Autodesk Fusion 360 part; units mm, degrees
(part 16 of 24)
  line L1627 (7.7089, 53.5468) -> (7.5354, 53.8714)
  line L1628 (4.6355, 51.6255) -> (4.6355, 48.2096)
  arc A4575 (6.3346, 55.2923) -> (6.1582, 55.0284) centre (6.2464, 55.1604) ccw
  line L1629 (6.2464, 55.1604) -> (5.9218, 55.3339)
  arc A4576 (7.8555, 53.6075) -> (7.5622, 53.486) centre (7.7088, 53.5468) ccw
  arc A4577 (7.22, 54.5627) -> (6.9746, 54.3613) centre (7.0973, 54.462) ccw
  line L1630 (5.9218, 55.3339) -> (5.5817, 55.4747)
  arc A4578 (5.6424, 55.6214) -> (5.5209, 55.3281) centre (5.5816, 55.4748) ccw
  arc A4579 (6.6407, 48.7982) -> (6.4643, 49.0621) centre (6.5525, 48.9301) ccw
  arc A4580 (7.4628, 54.2657) -> (7.1988, 54.0893) centre (7.3308, 54.1775) ccw
  arc A4581 (70.8706, 40.7824) -> (70.8706, 40.4649) centre (70.8706, 40.6237) ccw
  arc A4582 (70.2126, 40.4602) -> (70.4372, 40.2356) centre (70.3249, 40.3479) ccw
  arc A4583 (8.0017, 53.2528) -> (7.6978, 53.1606) centre (7.8497, 53.2067) ccw
  line L1631 (6.5525, 54.9558) -> (6.2464, 55.1604)
  line L1632 (7.5354, 53.8714) -> (7.3308, 54.1775)
  arc A4584 (7.8934, 52.2449) -> (8.2093, 52.2761) centre (8.0514, 52.2605) ccw
  arc A4585 (6.1582, 48.8576) -> (6.3346, 48.5936) centre (6.2464, 48.7256) ccw
  arc A4586 (72.0706, 39.9679) -> (72.2951, 40.1924) centre (72.1829, 40.0802) ccw
  arc A4587 (8.1123, 52.8854) -> (7.8009, 52.8235) centre (7.9566, 52.8545) ccw
  line L1633 (70.8706, 40.6237) -> (70.4098, 40.4328)
  arc A4588 (6.7363, 54.5996) -> (6.9377, 54.845) centre (6.837, 54.7223) ccw
  line L1634 (8.0284, 52.4934) -> (7.9566, 52.8544)
  arc A4589 (6.9377, 49.041) -> (6.7363, 49.2864) centre (6.837, 49.1637) ccw
  arc A4590 (70.5221, 40.3206) -> (70.2976, 40.5451) centre (70.4099, 40.4329) ccw
  arc A4591 (8.1864, 52.5089) -> (7.8704, 52.4778) centre (8.0284, 52.4934) ccw
  arc A4592 (7.5689, 53.4719) -> (7.8489, 53.6216) centre (7.7089, 53.5468) ccw
  arc A4593 (7.7031, 53.1459) -> (7.9964, 53.2674) centre (7.8498, 53.2067) ccw
  line L1635 (5.5817, 55.4747) -> (5.415, 55.5253)
  arc A4594 (6.9493, 54.8346) -> (6.7248, 54.6101) centre (6.8371, 54.7224) ccw
  arc A4595 (72.2149, 39.1206) -> (72.5324, 39.1206) centre (72.3736, 39.1206) ccw
  arc A4596 (5.9825, 48.4055) -> (5.861, 48.6988) centre (5.9218, 48.5522) ccw
  arc A4597 (7.8727, 52.4624) -> (8.1841, 52.5244) centre (8.0284, 52.4934) ccw
  arc A4598 (5.9966, 55.4739) -> (5.8469, 55.1939) centre (5.9217, 55.3339) ccw
  line L1636 (8.0514, 52.2605) -> (8.0284, 52.4934)
  arc A4599 (5.861, 55.1872) -> (5.9825, 55.4805) centre (5.9218, 55.3338) ccw
  arc A4600 (70.9314, 40.477) -> (70.8099, 40.7704) centre (70.8706, 40.6237) ccw
  line L1637 (5.415, 55.5253) -> (79.548, 55.5253)
  arc A4601 (5.5356, 55.3228) -> (5.6278, 55.6267) centre (5.5817, 55.4748) ccw
  arc A4602 (7.5622, 50.4) -> (7.8555, 50.2785) centre (7.7088, 50.3392) ccw
  line L1638 (71.3694, 40.6237) -> (70.8706, 40.6237)
  line L1639 (7.7089, 50.3392) -> (7.8497, 50.6793)
  line L1640 (7.3308, 54.1775) -> (7.0973, 54.462)
  line L1641 (72.3737, 39.1206) -> (72.3737, 39.6194)
  arc A4603 (72.5324, 39.6194) -> (72.2149, 39.6194) centre (72.3736, 39.6194) ccw
  line L1642 (6.5525, 48.9302) -> (6.837, 49.1637)
  arc A4604 (4.6355, 52.4192) -> (4.6355, 52.1017) centre (4.6355, 52.2604) ccw
  line L1643 (7.0973, 54.462) -> (6.837, 54.7223)
  arc A4605 (79.548, 55.3666) -> (79.548, 55.684) centre (79.548, 55.5253) ccw
  arc A4606 (7.1988, 49.7967) -> (7.4628, 49.6203) centre (7.3308, 49.7085) ccw
  line L1644 (72.3737, 39.6194) -> (72.1828, 40.0802)
  arc A4607 (7.8047, 52.8083) -> (8.1085, 52.9005) centre (7.9566, 52.8544) ccw
  arc A4608 (72.3295, 40.1409) -> (72.0362, 40.0194) centre (72.1829, 40.0802) ccw
  line L1645 (52.2859, 37.4845) -> (52.2859, 38.2029)
  arc A4609 (52.4446, 38.2029) -> (52.1271, 38.2029) centre (52.2858, 38.2029) ccw
  line L1646 (52.2859, 38.2029) -> (52.4751, 38.3921)
  arc A4610 (51.9362, 40.2012) -> (51.8147, 40.4946) centre (51.8755, 40.3479) ccw
  arc A4611 (50.0723, 36.5018) -> (50.2968, 36.7264) centre (50.1845, 36.6141) ccw
  arc A4612 (6.1716, 55.0203) -> (6.3212, 55.3004) centre (6.2464, 55.1604) ccw
  arc A4613 (71.7694, 40.2862) -> (71.8909, 40.5795) centre (71.8302, 40.4329) ccw
  arc A4614 (52.1271, 37.4845) -> (52.4446, 37.4845) centre (52.2858, 37.4845) ccw
  line L1647 (50.9029, 39.5859) -> (50.1845, 39.5859)
  line L1648 (52.4751, 38.3921) -> (70.3249, 38.3921)
  arc A4615 (70.3249, 38.2334) -> (70.3249, 38.5508) centre (70.3249, 38.3921) ccw
  arc A4616 (52.4751, 38.5508) -> (52.4751, 38.2334) centre (52.4751, 38.3921) ccw
  line L1649 (72.1828, 38.6598) -> (72.3737, 39.1206)
  line L1650 (71.3694, 38.1163) -> (71.8302, 38.3072)
  arc A4617 (50.1845, 36.7728) -> (50.1845, 36.4554) centre (50.1845, 36.6141) ccw
  arc A4618 (52.5873, 38.2798) -> (52.3628, 38.5044) centre (52.4751, 38.3921) ccw
  arc A4619 (52.3982, 37.3723) -> (52.1736, 37.5968) centre (52.2859, 37.4846) ccw
  arc A4620 (51.6283, 40.0868) -> (51.4038, 40.3113) centre (51.516, 40.199) ccw
  arc A4621 (52.1736, 38.3152) -> (52.3982, 38.0907) centre (52.2859, 38.203) ccw
  arc A4622 (70.4372, 38.5044) -> (70.2126, 38.2798) centre (70.3249, 38.3921) ccw
  arc A4623 (51.4155, 36.4554) -> (51.4155, 36.7728) centre (51.4155, 36.6141) ccw
  arc A4624 (49.4264, 37.5968) -> (49.2018, 37.3723) centre (49.3141, 37.4846) ccw
  line L1651 (70.4098, 38.3072) -> (70.8706, 38.1163)
  line L1652 (50.1845, 36.6141) -> (51.4155, 36.6141)
  arc A4625 (70.4706, 38.4538) -> (70.3491, 38.1605) centre (70.4099, 38.3072) ccw
  arc A4626 (70.8099, 37.9696) -> (70.9314, 38.263) centre (70.8706, 38.1163) ccw
  arc A4627 (50.7907, 39.6982) -> (51.0152, 39.4736) centre (50.903, 39.5859) ccw
  line L1653 (53.34, 17.78) -> (53.34, 19.2405)
  line L1654 (53.34, 19.2405) -> (53.34, 17.78)
  line L1655 (71.8302, 40.4328) -> (71.3694, 40.6237)
  line L1656 (51.5161, 40.199) -> (51.241, 39.9239)
  arc A4628 (71.4301, 40.7704) -> (71.3086, 40.477) centre (71.3693, 40.6237) ccw
  line L1657 (7.9566, 52.8544) -> (7.8497, 53.2067)
  arc A4629 (70.8706, 38.2751) -> (70.8706, 37.9576) centre (70.8706, 38.1164) ccw
  arc A4630 (72.2951, 38.5476) -> (72.0706, 38.7721) centre (72.1829, 38.6599) ccw
  line L1658 (51.8755, 40.3479) -> (51.5161, 40.199)
  line L1659 (70.8706, 38.1163) -> (71.3694, 38.1163)
  line L1660 (7.8497, 53.2067) -> (7.7089, 53.5468)
  arc A4631 (71.7179, 38.4194) -> (71.9424, 38.1949) centre (71.8302, 38.3072) ccw
  arc A4632 (49.2018, 38.8277) -> (49.4264, 38.6032) centre (49.3141, 38.7155) ccw
  arc A4633 (53.4988, 19.2405) -> (53.1813, 19.2405) centre (53.3401, 19.2405) ccw
  arc A4634 (70.3249, 40.1891) -> (70.3249, 40.5066) centre (70.3249, 40.3479) ccw
  arc A4635 (51.1287, 40.0362) -> (51.3532, 39.8117) centre (51.241, 39.924) ccw
  arc A4636 (71.3086, 38.263) -> (71.4301, 37.9696) centre (71.3693, 38.1163) ccw
  arc A4637 (50.9029, 39.4271) -> (50.9029, 39.7446) centre (50.9029, 39.5859) ccw
  arc A4638 (7.4034, 53.7832) -> (7.6673, 53.9596) centre (7.5353, 53.8714) ccw
  arc A4639 (51.3532, 39.8117) -> (51.1287, 40.0362) centre (51.241, 39.924) ccw
  arc A4640 (70.2976, 38.1949) -> (70.5221, 38.4194) centre (70.4099, 38.3072) ccw
  arc A4641 (7.2081, 54.0768) -> (7.4536, 54.2782) centre (7.3308, 54.1775) ccw
  arc A4642 (71.9424, 40.5451) -> (71.7179, 40.3206) centre (71.8302, 40.4328) ccw
  line L1661 (72.1828, 40.0802) -> (71.8302, 40.4328)
  arc A4643 (5.415, 55.684) -> (5.415, 55.3666) centre (5.415, 55.5253) ccw
  arc A4644 (51.8755, 40.5066) -> (51.8755, 40.1891) centre (51.8755, 40.3479) ccw
  arc A4645 (71.3694, 37.9576) -> (71.3694, 38.2751) centre (71.3694, 38.1164) ccw
  arc A4646 (6.9851, 54.3498) -> (7.2096, 54.5743) centre (7.0974, 54.4621) ccw
  line L1662 (49.3141, 37.4845) -> (50.1845, 36.6141)
  arc A4647 (50.2968, 39.4736) -> (50.0723, 39.6982) centre (50.1846, 39.5859) ccw
  arc A4648 (50.1845, 39.7446) -> (50.1845, 39.4271) centre (50.1845, 39.5859) ccw
  arc A4649 (51.3032, 36.7264) -> (51.5277, 36.5018) centre (51.4154, 36.6141) ccw
  arc A4650 (53.4987, 19.2405) -> (53.1812, 19.2405) centre (53.34, 19.2405) ccw
  line L1663 (70.3249, 40.3479) -> (51.8755, 40.3479)
  line L1664 (51.241, 39.9239) -> (50.9029, 39.5859)
  line L1665 (50.1845, 39.5859) -> (49.3141, 38.7155)
  arc A4651 (28.1833, 34.8511) -> (28.4079, 35.0756) centre (28.2956, 34.9634) ccw
  arc A4652 (53.945, 19.0817) -> (53.945, 19.3992) centre (53.945, 19.2405) ccw
  arc A4653 (53.34, 17.9388) -> (53.34, 17.6213) centre (53.34, 17.78) ccw
  line L1666 (49.3141, 38.7155) -> (49.3141, 37.4845)
  arc A4654 (16.5671, 14.6245) -> (16.8846, 14.6245) centre (16.7259, 14.6245) ccw
  line L1667 (25.0444, 37.4267) -> (25.6921, 36.779)
  line L1668 (27.3433, 39.7256) -> (25.9967, 39.7256)
  line L1669 (25.0444, 34.9633) -> (25.0444, 33.6167)
  arc A4655 (51.7104, 19.0868) -> (51.8319, 19.3801) centre (51.7712, 19.2334) ccw
  arc A4656 (27.4891, 35.611) -> (27.8066, 35.611) centre (27.6479, 35.611) ccw
  arc A4657 (28.4543, 34.9633) -> (28.1368, 34.9633) centre (28.2956, 34.9633) ccw
  line L1670 (70.3249, 38.3921) -> (70.4098, 38.3072)
  arc A4658 (25.5798, 36.6667) -> (25.8044, 36.8912) centre (25.6921, 36.779) ccw
  line L1671 (52.2496, 18.7551) -> (51.7712, 19.2335)
  line L1672 (50.459, 19.4945) -> (49.8288, 19.2335)
  line L1673 (52.735, 19.2405) -> (52.2496, 18.7551)
  arc A4659 (46.4368, 21.5237) -> (46.6613, 21.7482) centre (46.549, 21.636) ccw
  arc A4660 (27.3433, 39.5668) -> (27.3433, 39.8843) centre (27.3433, 39.7256) ccw
  arc A4661 (72.0362, 38.7206) -> (72.3295, 38.5991) centre (72.1829, 38.6599) ccw
  arc A4662 (46.2739, 22.0698) -> (46.2739, 21.7523) centre (46.2739, 21.9111) ccw
  arc A4663 (25.5333, 35.611) -> (25.8509, 35.611) centre (25.6921, 35.611) ccw
  line L1674 (25.6921, 36.779) -> (25.6921, 35.611)
  line L1675 (28.2956, 38.7733) -> (27.3433, 39.7256)
  arc A4664 (25.8044, 35.4988) -> (25.5798, 35.7233) centre (25.6921, 35.6111) ccw
  arc A4665 (28.1368, 37.4267) -> (28.4543, 37.4267) centre (28.2956, 37.4267) ccw
  arc A4666 (24.8856, 33.6167) -> (25.2032, 33.6167) centre (25.0444, 33.6167) ccw
  arc A4667 (72.5204, 39.0599) -> (72.227, 39.1814) centre (72.3737, 39.1206) ccw
  arc A4668 (50.459, 19.6532) -> (50.459, 19.3357) centre (50.459, 19.4945) ccw
  arc A4669 (51.141, 19.3357) -> (51.141, 19.6532) centre (51.141, 19.4945) ccw
  arc A4670 (51.8834, 19.3457) -> (51.6589, 19.1212) centre (51.7712, 19.2335) ccw
  line L1676 (27.3433, 32.6644) -> (28.2956, 33.6167)
  arc A4671 (27.2311, 32.7767) -> (27.4556, 32.5521) centre (27.3434, 32.6644) ccw
  arc A4672 (28.1368, 33.6167) -> (28.4543, 33.6167) centre (28.2956, 33.6167) ccw
  arc A4673 (52.1373, 18.6428) -> (52.3619, 18.8673) centre (52.2496, 18.755) ccw
  arc A4674 (49.7681, 19.3801) -> (49.8896, 19.0868) centre (49.8289, 19.2335) ccw
  arc A4675 (50.5197, 19.3478) -> (50.3982, 19.6412) centre (50.459, 19.4945) ccw
  line L1677 (51.7712, 19.2335) -> (51.141, 19.4945)
  arc A4676 (52.735, 19.3992) -> (52.735, 19.0817) centre (52.735, 19.2405) ccw
  arc A4677 (51.2018, 19.6412) -> (51.0803, 19.3478) centre (51.1411, 19.4945) ccw
  line L1678 (71.8302, 38.3072) -> (72.1828, 38.6598)
  arc A4678 (49.1554, 37.4845) -> (49.4729, 37.4845) centre (49.3142, 37.4845) ccw
  arc A4679 (27.8066, 36.779) -> (27.4891, 36.779) centre (27.6479, 36.779) ccw
  line L1679 (27.6479, 36.779) -> (28.2956, 37.4267)
  line L1680 (51.141, 19.4945) -> (50.459, 19.4945)
  arc A4680 (52.8473, 19.1282) -> (52.6228, 19.3528) centre (52.7351, 19.2405) ccw
  arc A4681 (53.1813, 17.78) -> (53.4988, 17.78) centre (53.3401, 17.78) ccw
  line L1681 (51.4155, 36.6141) -> (52.2859, 37.4845)
  arc A4682 (53.34, 19.0817) -> (53.34, 19.3992) centre (53.34, 19.2405) ccw
  arc A4683 (71.8909, 38.1605) -> (71.7694, 38.4538) centre (71.8302, 38.3072) ccw
  arc A4684 (52.1373, 18.8673) -> (52.3619, 18.6428) centre (52.2496, 18.7551) ccw
  line L1682 (53.34, 19.2405) -> (52.735, 19.2405)
  arc A4685 (53.1812, 17.78) -> (53.4987, 17.78) centre (53.34, 17.78) ccw
  arc A4686 (27.4556, 39.8379) -> (27.2311, 39.6133) centre (27.3434, 39.7256) ccw
  arc A4687 (12.7062, 34.7907) -> (12.4129, 34.9122) centre (12.5596, 34.8514) ccw
  arc A4688 (49.4729, 38.7155) -> (49.1554, 38.7155) centre (49.3142, 38.7155) ccw
  arc A4689 (14.6245, 16.8846) -> (14.6245, 16.5671) centre (14.6245, 16.7259) ccw
  arc A4690 (51.4553, 40.3457) -> (51.5768, 40.0524) centre (51.516, 40.1991) ccw
  arc A4691 (53.34, 17.6213) -> (53.34, 17.9388) centre (53.34, 17.78) ccw
  line L1683 (25.9967, 32.6644) -> (27.3433, 32.6644)
  line L1684 (15.8555, 16.7259) -> (14.6245, 16.7259)
  arc A4692 (14.7368, 16.6136) -> (14.5123, 16.8382) centre (14.6245, 16.7259) ccw
  arc A4693 (15.9677, 16.8382) -> (15.7432, 16.6136) centre (15.8555, 16.7259) ccw
  arc A4694 (16.8846, 15.8555) -> (16.5671, 15.8555) centre (16.7259, 15.8555) ccw
  line L1685 (7.62, 21.59) -> (7.62, 23.4315)
  line L1686 (14.6245, 16.7259) -> (13.7541, 15.8555)
  arc A4695 (7.7787, 21.59) -> (7.4612, 21.59) centre (7.62, 21.59) ccw
  line L1687 (13.7541, 15.8555) -> (13.7541, 14.6245)
  line L1688 (5.7785, 22.3528) -> (5.7785, 21.59)
  arc A4696 (13.6418, 15.9677) -> (13.8664, 15.7432) centre (13.7541, 15.8554) ccw
  arc A4697 (28.1833, 38.6611) -> (28.4079, 38.8856) centre (28.2956, 38.7734) ccw
  arc A4698 (15.8555, 13.5954) -> (15.8555, 13.9129) centre (15.8555, 13.7542) ccw
  arc A4699 (9.3027, 20.8272) -> (9.6202, 20.8272) centre (9.4615, 20.8272) ccw
  line L1689 (6.8572, 23.4315) -> (5.7785, 22.3528)
  line L1690 (25.9967, 39.7256) -> (25.0444, 38.7733)
  arc A4700 (25.9967, 39.8843) -> (25.9967, 39.5668) centre (25.9967, 39.7256) ccw
  line L1691 (25.0444, 38.7733) -> (25.0444, 37.4267)
  arc A4701 (25.1567, 33.7289) -> (24.9321, 33.5044) centre (25.0444, 33.6167) ccw
  arc A4702 (7.62, 21.4312) -> (7.62, 21.7487) centre (7.62, 21.59) ccw
  arc A4703 (25.8509, 36.779) -> (25.5333, 36.779) centre (25.6921, 36.779) ccw
  arc A4704 (25.8844, 32.5521) -> (26.1089, 32.7767) centre (25.9966, 32.6644) ccw
  arc A4705 (28.4079, 37.3144) -> (28.1833, 37.5389) centre (28.2956, 37.4267) ccw
  arc A4706 (24.9321, 38.8856) -> (25.1567, 38.6611) centre (25.0444, 38.7734) ccw
  arc A4707 (28.4543, 38.7733) -> (28.1368, 38.7733) centre (28.2956, 38.7733) ccw
  line L1692 (25.6921, 35.611) -> (25.0444, 34.9633)
  arc A4708 (26.1089, 39.6133) -> (25.8844, 39.8379) centre (25.9966, 39.7256) ccw
  arc A4709 (27.3433, 32.5057) -> (27.3433, 32.8231) centre (27.3433, 32.6644) ccw
  arc A4710 (25.2032, 34.9633) -> (24.8856, 34.9633) centre (25.0444, 34.9633) ccw
  line L1693 (27.6479, 35.611) -> (27.6479, 36.779)
  arc A4711 (16.6136, 15.7432) -> (16.8382, 15.9677) centre (16.7259, 15.8554) ccw
  arc A4712 (25.9967, 32.8231) -> (25.9967, 32.5057) centre (25.9967, 32.6644) ccw
  line L1694 (28.2956, 33.6167) -> (28.2956, 34.9633)
  line L1695 (16.7259, 14.6245) -> (16.7259, 15.8555)
  arc A4713 (27.7602, 35.7233) -> (27.5356, 35.4988) centre (27.6479, 35.611) ccw
  arc A4714 (24.9321, 35.0756) -> (25.1567, 34.8511) centre (25.0444, 34.9634) ccw
  line L1696 (16.7259, 15.8555) -> (15.8555, 16.7259)
  line L1697 (28.2956, 37.4267) -> (28.2956, 38.7733)
  arc A4715 (25.2032, 38.7733) -> (24.8856, 38.7733) centre (25.0444, 38.7733) ccw
  arc A4716 (24.8856, 37.4267) -> (25.2032, 37.4267) centre (25.0444, 37.4267) ccw
  arc A4717 (13.8664, 14.7368) -> (13.6418, 14.5123) centre (13.7541, 14.6246) ccw
  arc A4718 (7.4612, 19.7485) -> (7.7787, 19.7485) centre (7.62, 19.7485) ccw
  line L1698 (9.4615, 21.59) -> (9.4615, 22.3528)
  arc A4719 (5.6662, 22.465) -> (5.8908, 22.2405) centre (5.7785, 22.3528) ccw
  arc A4720 (25.1567, 37.5389) -> (24.9321, 37.3144) centre (25.0444, 37.4267) ccw
  arc A4721 (6.9695, 23.3192) -> (6.745, 23.5438) centre (6.8573, 23.4315) ccw
  arc A4722 (28.4079, 33.5044) -> (28.1833, 33.7289) centre (28.2956, 33.6167) ccw
  line L1699 (25.0444, 33.6167) -> (25.9967, 32.6644)
  line L1700 (14.6245, 13.7541) -> (15.8555, 13.7541)
  arc A4723 (7.4612, 21.59) -> (7.7787, 21.59) centre (7.62, 21.59) ccw
  line L1701 (7.62, 19.7485) -> (8.3828, 19.7485)
  arc A4724 (7.62, 21.7488) -> (7.62, 21.4313) centre (7.62, 21.5901) ccw
  arc A4725 (27.5356, 36.8912) -> (27.7602, 36.6667) centre (27.6479, 36.7789) ccw
  arc A4726 (7.7788, 23.4315) -> (7.4613, 23.4315) centre (7.6201, 23.4315) ccw
  arc A4727 (6.8572, 19.9073) -> (6.8572, 19.5897) centre (6.8572, 19.7485) ccw
  line L1702 (7.62, 21.59) -> (9.4615, 21.59)
  line L1703 (8.3828, 19.7485) -> (9.4615, 20.8272)
  line L1704 (28.2956, 34.9633) -> (27.6479, 35.611)
  arc A4728 (15.8555, 16.5671) -> (15.8555, 16.8846) centre (15.8555, 16.7259) ccw
  line L1705 (9.4615, 20.8272) -> (9.4615, 21.59)
  arc A4729 (8.495, 23.5438) -> (8.2705, 23.3192) centre (8.3827, 23.4315) ccw
  arc A4730 (14.5123, 13.6418) -> (14.7368, 13.8664) centre (14.6246, 13.7541) ccw
  arc A4731 (7.4613, 21.59) -> (7.7788, 21.59) centre (7.6201, 21.59) ccw
  arc A4732 (9.4615, 21.4312) -> (9.4615, 21.7487) centre (9.4615, 21.59) ccw
  arc A4733 (15.7432, 13.8664) -> (15.9677, 13.6418) centre (15.8554, 13.7541) ccw
  line L1706 (15.2918, 24.8452) -> (15.7526, 24.6543)
  arc A4734 (7.4613, 19.7485) -> (7.7788, 19.7485) centre (7.6201, 19.7485) ccw
  line L1707 (14.7483, 26.1574) -> (14.7483, 25.6586)
  line L1708 (13.7541, 14.6245) -> (14.6245, 13.7541)
  arc A4735 (7.62, 21.4313) -> (7.62, 21.7488) centre (7.62, 21.5901) ccw
  arc A4736 (8.2705, 19.8608) -> (8.495, 19.6362) centre (8.3827, 19.7485) ccw
  line L1709 (9.4615, 21.59) -> (7.62, 21.59)
  arc A4737 (7.62, 23.2727) -> (7.62, 23.5902) centre (7.62, 23.4315) ccw
  arc A4738 (7.62, 21.4312) -> (7.62, 21.7487) centre (7.62, 21.59) ccw
  arc A4739 (15.7526, 24.8131) -> (15.7526, 24.4956) centre (15.7526, 24.6543) ccw
  arc A4740 (5.7785, 21.7488) -> (5.7785, 21.4313) centre (5.7785, 21.5901) ccw
  arc A4741 (7.4613, 21.59) -> (7.7788, 21.59) centre (7.6201, 21.59) ccw
  arc A4742 (5.6197, 21.59) -> (5.9373, 21.59) centre (5.7785, 21.59) ccw
  line L1710 (8.6955, 26.9621) -> (15.2831, 26.9621)
  arc A4743 (13.9129, 15.8555) -> (13.5954, 15.8555) centre (13.7542, 15.8555) ccw
  arc A4744 (7.62, 21.7488) -> (7.62, 21.4313) centre (7.62, 21.5901) ccw
  arc A4745 (7.62, 21.7487) -> (7.62, 21.4312) centre (7.62, 21.59) ccw
  arc A4746 (7.7788, 21.59) -> (7.4613, 21.59) centre (7.6201, 21.59) ccw
  arc A4747 (9.3027, 21.59) -> (9.6202, 21.59) centre (9.4615, 21.59) ccw
  line L1711 (8.488, 31.3055) -> (6.752, 31.3055)
  arc A4748 (9.3492, 22.2405) -> (9.5738, 22.465) centre (9.4615, 22.3527) ccw
  arc A4749 (5.4122, 30.1902) -> (5.6368, 29.9657) centre (5.5245, 30.078) ccw
  arc A4750 (9.6032, 29.9657) -> (9.8278, 30.1902) centre (9.7155, 30.078) ccw
  arc A4751 (8.3828, 23.2727) -> (8.3828, 23.5902) centre (8.3828, 23.4315) ccw
  arc A4752 (7.62, 19.9073) -> (7.62, 19.5897) centre (7.62, 19.7485) ccw
  arc A4753 (9.5738, 20.715) -> (9.3492, 20.9395) centre (9.4615, 20.8272) ccw
  line L1712 (7.62, 19.7485) -> (7.62, 21.59)
  line L1713 (7.62, 23.4315) -> (6.8572, 23.4315)
  arc A4754 (8.4448, 27.2267) -> (8.2202, 27.0023) centre (8.3325, 27.1145) ccw
  arc A4755 (7.62, 21.7487) -> (7.62, 21.4312) centre (7.62, 21.59) ccw
  line L1714 (15.7526, 24.6543) -> (16.2514, 24.6543)
  arc A4756 (8.3968, 27.2576) -> (8.2753, 26.9643) centre (8.3361, 27.111) ccw
  line L1715 (8.3828, 23.4315) -> (7.62, 23.4315)
  arc A4757 (6.8572, 23.5902) -> (6.8572, 23.2727) centre (6.8572, 23.4315) ccw
  arc A4758 (8.3325, 26.9557) -> (8.3325, 27.2733) centre (8.3325, 27.1145) ccw
  line L1716 (7.62, 21.59) -> (7.62, 19.7485)
  arc A4759 (9.4615, 21.4313) -> (9.4615, 21.7488) centre (9.4615, 21.5901) ccw
  arc A4760 (7.62, 19.5897) -> (7.62, 19.9073) centre (7.62, 19.7485) ccw
  arc A4761 (9.6202, 22.3528) -> (9.3027, 22.3528) centre (9.4615, 22.3528) ccw
  arc A4762 (16.8382, 14.5123) -> (16.6136, 14.7368) centre (16.7259, 14.6246) ccw
  arc A4763 (14.6016, 26.2181) -> (14.895, 26.0966) centre (14.7483, 26.1574) ccw
  arc A4764 (16.2514, 24.4956) -> (16.2514, 24.8131) centre (16.2514, 24.6543) ccw
  arc A4765 (6.752, 31.4642) -> (6.752, 31.1467) centre (6.752, 31.3054) ccw
  line L1717 (6.8572, 19.7485) -> (7.62, 19.7485)
  arc A4766 (14.6245, 13.9129) -> (14.6245, 13.5954) centre (14.6245, 13.7542) ccw
  arc A4767 (13.5954, 14.6245) -> (13.9129, 14.6245) centre (13.7542, 14.6245) ccw
  arc A4768 (15.0514, 25.3101) -> (14.8269, 25.0856) centre (14.9391, 25.1979) ccw
  arc A4769 (15.3954, 26.8498) -> (15.1709, 27.0744) centre (15.2831, 26.9621) ccw
  arc A4770 (7.62, 23.5902) -> (7.62, 23.2727) centre (7.62, 23.4315) ccw
  line L1718 (9.4615, 22.3528) -> (8.3828, 23.4315)
  arc A4771 (6.8643, 31.1932) -> (6.6398, 31.4178) centre (6.7521, 31.3055) ccw
  arc A4772 (8.3828, 19.5897) -> (8.3828, 19.9073) centre (8.3828, 19.7485) ccw
  arc A4773 (7.7788, 21.59) -> (7.4613, 21.59) centre (7.6201, 21.59) ccw
  arc A4774 (15.3526, 24.9918) -> (15.2311, 24.6985) centre (15.2918, 24.8452) ccw
  arc A4775 (14.8269, 26.7304) -> (15.0514, 26.5059) centre (14.9391, 26.6182) ccw
  line L1719 (14.9392, 25.1978) -> (15.2918, 24.8452)
  arc A4776 (8.6955, 27.1209) -> (8.6955, 26.8034) centre (8.6955, 26.9622) ccw
  arc A4777 (9.6202, 21.59) -> (9.3027, 21.59) centre (9.4615, 21.59) ccw
  line L1720 (7.62, 23.4315) -> (7.62, 21.59)
  arc A4778 (15.0858, 26.5574) -> (14.7925, 26.6789) centre (14.9392, 26.6181) ccw
  line L1721 (15.8555, 13.7541) -> (16.7259, 14.6245)
  line L1722 (8.3325, 27.1145) -> (8.3361, 27.111)
  arc A4779 (7.7787, 23.4315) -> (7.4612, 23.4315) centre (7.62, 23.4315) ccw
  arc A4780 (5.7785, 21.7487) -> (5.7785, 21.4312) centre (5.7785, 21.59) ccw
  arc A4781 (14.895, 25.7194) -> (14.6016, 25.5979) centre (14.7483, 25.6587) ccw
  arc A4782 (5.8908, 20.9395) -> (5.6662, 20.715) centre (5.7785, 20.8272) ccw
  line L1723 (5.7785, 21.59) -> (7.62, 21.59)
  arc A4783 (14.5896, 25.6586) -> (14.907, 25.6586) centre (14.7483, 25.6586) ccw
  line L1724 (8.3361, 27.111) -> (8.6955, 26.9621)
  line L1725 (5.7785, 20.8272) -> (6.8572, 19.7485)
  arc A4784 (7.7787, 21.59) -> (7.4612, 21.59) centre (7.62, 21.59) ccw
  arc A4785 (7.4612, 21.59) -> (7.7787, 21.59) centre (7.62, 21.59) ccw
  arc A4786 (5.6197, 20.8272) -> (5.9373, 20.8272) centre (5.7785, 20.8272) ccw
  line L1726 (5.7785, 21.59) -> (5.7785, 20.8272)
  arc A4787 (6.752, 27.2733) -> (6.752, 26.9557) centre (6.752, 27.1145) ccw
  arc A4788 (8.488, 31.1467) -> (8.488, 31.4642) centre (8.488, 31.3054) ccw
  arc A4789 (8.6347, 26.8154) -> (8.7562, 27.1088) centre (8.6955, 26.9621) ccw
  line L1727 (16.2514, 24.6543) -> (16.5186, 24.765)
  arc A4790 (5.9373, 22.3528) -> (5.6197, 22.3528) centre (5.7785, 22.3528) ccw
  line L1728 (6.752, 31.3055) -> (5.5245, 30.078)
  line L1729 (28.1196, 23.4133) -> (28.2255, 23.3074)
  line L1730 (27.0211, 22.6949) -> (27.67, 22.9637)
  line L1731 (29.21, 25.4) -> (29.21, 22.9489)
  arc A4791 (16.5186, 24.9238) -> (16.5186, 24.6062) centre (16.5186, 24.765) ccw
  arc A4792 (8.2238, 26.9988) -> (8.4484, 27.2232) centre (8.3361, 27.111) ccw
  line L1732 (28.6299, 23.0596) -> (28.8561, 22.9861)
  line L1733 (9.7155, 30.078) -> (8.488, 31.3055)
  arc A4793 (29.21, 22.7902) -> (29.21, 23.1077) centre (29.21, 22.9489) ccw
  arc A4794 (15.6919, 24.5076) -> (15.8134, 24.801) centre (15.7527, 24.6543) ccw
  line L1734 (15.2831, 26.9621) -> (14.9392, 26.6182)
  arc A4795 (25.0514, 24.1698) -> (24.758, 24.0483) centre (24.9047, 24.109) ccw
  line L1735 (20.9425, 24.431) -> (21.3626, 24.257)
  arc A4796 (28.2319, 23.5255) -> (28.0073, 23.301) centre (28.1196, 23.4133) ccw
  line L1736 (6.752, 27.1145) -> (8.3325, 27.1145)
  line L1737 (5.5245, 28.342) -> (6.752, 27.1145)
  arc A4797 (28.1132, 23.1952) -> (28.3377, 23.4197) centre (28.2255, 23.3075) ccw
  arc A4798 (6.745, 19.6362) -> (6.9695, 19.8608) centre (6.8573, 19.7485) ccw
  arc A4799 (28.3246, 23.0392) -> (28.5112, 23.296) centre (28.4179, 23.1676) ccw
  line L1738 (20.6086, 24.765) -> (20.621, 24.7525)
  line L1739 (29.21, 22.9489) -> (29.21, 25.4)
  arc A4800 (16.5794, 24.6183) -> (16.4579, 24.9117) centre (16.5187, 24.765) ccw
  arc A4801 (16.1906, 24.801) -> (16.3121, 24.5076) centre (16.2514, 24.6543) ccw
  arc A4802 (24.9047, 24.0983) -> (24.9047, 24.4158) centre (24.9047, 24.2571) ccw
  line L1740 (28.4179, 23.1676) -> (28.6299, 23.0596)
  line L1741 (16.5186, 24.765) -> (20.6086, 24.765)
  arc A4803 (29.0662, 22.7921) -> (29.1159, 23.1057) centre (29.0911, 22.9489) ccw
  arc A4804 (6.6398, 27.0022) -> (6.8643, 27.2268) centre (6.7521, 27.1145) ccw
  arc A4805 (25.0268, 23.3995) -> (25.3201, 23.521) centre (25.1735, 23.4603) ccw
  arc A4806 (14.907, 26.1574) -> (14.5896, 26.1574) centre (14.7483, 26.1574) ccw
  line L1742 (20.621, 24.7525) -> (20.9425, 24.431)
  arc A4807 (5.6833, 30.078) -> (5.3658, 30.078) centre (5.5246, 30.078) ccw
  arc A4808 (5.9373, 21.59) -> (5.6197, 21.59) centre (5.7785, 21.59) ccw
  line L1743 (14.9392, 26.6182) -> (14.7483, 26.1574)
  arc A4809 (14.7925, 25.1371) -> (15.0858, 25.2586) centre (14.9392, 25.1979) ccw
  line L1744 (7.62, 21.59) -> (5.7785, 21.59)
  arc A4810 (7.62, 21.4313) -> (7.62, 21.7488) centre (7.62, 21.5901) ccw
  arc A4811 (5.6368, 28.4543) -> (5.4122, 28.2298) centre (5.5245, 28.3421) ccw
  arc A4812 (15.1796, 24.7329) -> (15.4041, 24.9574) centre (15.2919, 24.8452) ccw
  arc A4813 (15.2831, 26.8034) -> (15.2831, 27.1209) centre (15.2831, 26.9622) ccw
  line L1745 (5.5245, 30.078) -> (5.5245, 28.342)
  line L1746 (14.7483, 25.6586) -> (14.9392, 25.1978)
  arc A4814 (8.6002, 31.4178) -> (8.3757, 31.1932) centre (8.4879, 31.3055) ccw
  arc A4815 (5.3658, 28.342) -> (5.6833, 28.342) centre (5.5246, 28.342) ccw
  line L1747 (24.9047, 24.257) -> (24.9047, 24.1091)
  arc A4816 (21.3019, 24.1103) -> (21.4234, 24.4037) centre (21.3627, 24.257) ccw
  line L1748 (30.3004, 23.4133) -> (30.75, 22.9637)
  line L1749 (25.67, 22.9637) -> (26.3189, 22.6949)
  line L1750 (21.3626, 24.257) -> (24.9047, 24.257)
  arc A4817 (27.0211, 22.5361) -> (27.0211, 22.8537) centre (27.0211, 22.6949) ccw
  arc A4818 (28.8809, 23.1429) -> (28.8313, 22.8293) centre (28.8561, 22.9861) ccw
  arc A4819 (29.0513, 22.9489) -> (29.3688, 22.9489) centre (29.2101, 22.9489) ccw
  arc A4820 (24.746, 24.1091) -> (25.0635, 24.1091) centre (24.9048, 24.1091) ccw
  line L1751 (25.1735, 23.4602) -> (25.67, 22.9637)
  arc A4821 (21.0033, 24.5777) -> (20.8818, 24.2843) centre (20.9426, 24.431) ccw
  arc A4822 (25.0635, 24.257) -> (24.746, 24.257) centre (24.9048, 24.257) ccw
  arc A4823 (28.6789, 23.2106) -> (28.5808, 22.9086) centre (28.6298, 23.0596) ccw
  arc A4824 (25.2857, 23.5725) -> (25.0612, 23.348) centre (25.1735, 23.4603) ccw
  arc A4825 (28.5578, 22.9182) -> (28.7019, 23.2011) centre (28.6299, 23.0597) ccw
  line L1752 (35.29, 22.9637) -> (35.56, 23.2337)
  arc A4826 (29.21, 25.2412) -> (29.21, 25.5587) centre (29.21, 25.4) ccw
  arc A4827 (20.7333, 24.8648) -> (20.5088, 24.6403) centre (20.621, 24.7526) ccw
  arc A4828 (29.0512, 22.9489) -> (29.3687, 22.9489) centre (29.2099, 22.9489) ccw
  line L1753 (28.8561, 22.9861) -> (29.0911, 22.9489)
  line L1754 (28.2255, 23.3074) -> (28.4179, 23.1676)
  arc A4829 (35.1777, 23.0759) -> (35.4022, 22.8514) centre (35.29, 22.9637) ccw
  arc A4830 (25.7308, 23.1103) -> (25.6093, 22.817) centre (25.67, 22.9637) ccw
  line L1755 (37.1811, 22.6949) -> (37.83, 22.9637)
  arc A4831 (29.9088, 23.296) -> (30.0954, 23.0392) centre (30.0021, 23.1676) ccw
  arc A4832 (28.3188, 23.4359) -> (28.1321, 23.179) centre (28.2254, 23.3075) ccw
  arc A4833 (29.3687, 25.4) -> (29.0512, 25.4) centre (29.2099, 25.4) ccw
  arc A4834 (26.3189, 22.8537) -> (26.3189, 22.5361) centre (26.3189, 22.6949) ccw
  arc A4835 (20.8303, 24.3188) -> (21.0548, 24.5433) centre (20.9426, 24.431) ccw
  arc A4836 (25.5578, 22.8514) -> (25.7823, 23.0759) centre (25.67, 22.9637) ccw
  line L1756 (26.3189, 22.6949) -> (27.0211, 22.6949)
  arc A4837 (26.9604, 22.8416) -> (27.0819, 22.5482) centre (27.0211, 22.6949) ccw
  arc A4838 (21.3626, 24.4158) -> (21.3626, 24.0983) centre (21.3626, 24.2571) ccw
  line L1757 (27.67, 22.9637) -> (28.1196, 23.4133)
  arc A4839 (28.807, 22.8351) -> (28.9052, 23.1371) centre (28.8561, 22.9861) ccw
  line L1758 (33.29, 22.9637) -> (33.9389, 22.6949)
  arc A4840 (35.8908, 23.1103) -> (35.7693, 22.817) centre (35.83, 22.9637) ccw
  arc A4841 (29.0911, 23.1077) -> (29.0911, 22.7902) centre (29.0911, 22.9489) ccw
  arc A4842 (29.21, 25.5587) -> (29.21, 25.2412) centre (29.21, 25.4) ccw
  arc A4843 (27.5577, 23.0759) -> (27.7822, 22.8514) centre (27.67, 22.9637) ccw
  line L1759 (24.9047, 24.1091) -> (25.1735, 23.4602)
  arc A4844 (32.8107, 22.817) -> (32.6892, 23.1103) centre (32.7499, 22.9637) ccw
  arc A4845 (37.1811, 22.5361) -> (37.1811, 22.8537) centre (37.1811, 22.6949) ccw
  arc A4846 (29.5887, 22.8293) -> (29.5391, 23.1429) centre (29.5639, 22.9861) ccw
  arc A4847 (29.3041, 23.1057) -> (29.3538, 22.7921) centre (29.329, 22.9489) ccw
  arc A4848 (35.3507, 22.817) -> (35.2292, 23.1103) centre (35.29, 22.9637) ccw
  arc A4849 (28.49, 23.3091) -> (28.3458, 23.0262) centre (28.4179, 23.1677) ccw
  arc A4850 (30.6378, 22.8514) -> (30.8623, 23.0759) centre (30.7501, 22.9637) ccw
  line L1760 (32.75, 22.9637) -> (33.02, 23.2337)
  line L1761 (33.9389, 22.6949) -> (34.6411, 22.6949)
  arc A4851 (28.2319, 23.301) -> (28.0073, 23.5255) centre (28.1196, 23.4133) ccw
  arc A4852 (20.6086, 24.6062) -> (20.6086, 24.9238) centre (20.6086, 24.765) ccw
  arc A4853 (31.3381, 22.5482) -> (31.4596, 22.8416) centre (31.3989, 22.6949) ccw
  arc A4854 (26.2581, 22.5482) -> (26.3796, 22.8416) centre (26.3189, 22.6949) ccw
  arc A4855 (20.5088, 24.6403) -> (20.7333, 24.8648) centre (20.621, 24.7526) ccw
  line L1762 (30.75, 22.9637) -> (31.3989, 22.6949)
  arc A4856 (32.0404, 22.8416) -> (32.1619, 22.5482) centre (32.1012, 22.6949) ccw
  line L1763 (30.1945, 23.3074) -> (30.3004, 23.4133)
  arc A4857 (32.6377, 23.0759) -> (32.8622, 22.8514) centre (32.75, 22.9637) ccw
  line L1764 (29.5639, 22.9861) -> (29.7901, 23.0596)
  arc A4858 (34.6411, 22.5361) -> (34.6411, 22.8537) centre (34.6411, 22.6949) ccw
  arc A4859 (37.8907, 22.817) -> (37.7692, 23.1103) centre (37.83, 22.9637) ccw
  arc A4860 (20.7208, 24.8773) -> (20.4963, 24.6527) centre (20.6086, 24.765) ccw
  arc A4861 (27.7307, 22.817) -> (27.6092, 23.1103) centre (27.67, 22.9637) ccw
  line L1765 (29.0911, 22.9489) -> (29.21, 22.9489)
  arc A4862 (35.6723, 23.1214) -> (35.4477, 23.3459) centre (35.56, 23.2336) ccw
  line L1766 (33.9389, 28.1051) -> (33.29, 27.8363)
  arc A4863 (36.5396, 27.9584) -> (36.4181, 28.2518) centre (36.4789, 28.1051) ccw
  arc A4864 (38.4388, 23.348) -> (38.2143, 23.5725) centre (38.3266, 23.4603) ccw
  arc A4865 (33.9389, 22.8537) -> (33.9389, 22.5361) centre (33.9389, 22.6949) ccw
  arc A4866 (30.2879, 23.179) -> (30.1012, 23.4359) centre (30.1946, 23.3075) ccw
  arc A4867 (36.4181, 22.5482) -> (36.5396, 22.8416) centre (36.4789, 22.6949) ccw
  arc A4868 (31.3989, 22.8537) -> (31.3989, 22.5361) centre (31.3989, 22.6949) ccw
  arc A4869 (30.4126, 23.301) -> (30.1881, 23.5255) centre (30.3004, 23.4133) ccw
  arc A4870 (32.9077, 27.4541) -> (33.1323, 27.6786) centre (33.02, 27.5663) ccw
  arc A4871 (33.4023, 27.7241) -> (33.1778, 27.9486) centre (33.2901, 27.8364) ccw
  arc A4872 (35.2292, 27.6897) -> (35.3507, 27.983) centre (35.29, 27.8364) ccw
  line L1767 (34.6411, 22.6949) -> (35.29, 22.9637)
  arc A4873 (33.1323, 23.1214) -> (32.9077, 23.3459) centre (33.02, 23.2336) ccw
  arc A4874 (33.3508, 23.1103) -> (33.2293, 22.817) centre (33.2901, 22.9636) ccw
  arc A4875 (35.4477, 27.4541) -> (35.6723, 27.6786) centre (35.56, 27.5663) ccw
  arc A4876 (29.93, 27.4909) -> (30.0742, 27.7738) centre (30.0021, 27.6324) ccw
  line L1768 (38.5953, 24.1091) -> (38.5953, 26.6909)
  arc A4877 (37.1811, 27.9463) -> (37.1811, 28.2638) centre (37.1811, 28.1051) ccw
  line L1769 (33.29, 27.8363) -> (33.02, 27.5663)
  line L1770 (31.3989, 22.6949) -> (32.1011, 22.6949)
  line L1771 (35.56, 23.2337) -> (35.83, 22.9637)
  arc A4878 (33.9389, 28.2638) -> (33.9389, 27.9463) centre (33.9389, 28.1051) ccw
  arc A4879 (32.8622, 27.9486) -> (32.6377, 27.7241) centre (32.75, 27.8364) ccw
  arc A4880 (30.0954, 27.7608) -> (29.9088, 27.5039) centre (30.0021, 27.6324) ccw
  line L1772 (30.0021, 23.1676) -> (30.1945, 23.3074)
  arc A4881 (30.4126, 23.5255) -> (30.1881, 23.301) centre (30.3004, 23.4133) ccw
  arc A4882 (30.0742, 23.0262) -> (29.93, 23.3091) centre (30.0021, 23.1676) ccw
  arc A4883 (34.5804, 22.8416) -> (34.7019, 22.5482) centre (34.6412, 22.6949) ccw
  line L1773 (36.4789, 28.1051) -> (35.83, 27.8363)
  line L1774 (38.3265, 27.3398) -> (37.83, 27.8363)
  arc A4884 (37.1204, 22.8416) -> (37.2419, 22.5482) centre (37.1812, 22.6949) ccw
  arc A4885 (29.3289, 22.7902) -> (29.3289, 23.1077) centre (29.3289, 22.9489) ccw
  line L1775 (33.02, 23.2337) -> (33.29, 22.9637)
  arc A4886 (29.7181, 23.2011) -> (29.8622, 22.9182) centre (29.7902, 23.0597) ccw
  line L1776 (30.0021, 27.6324) -> (29.7901, 27.7404)
  arc A4887 (30.0823, 23.4197) -> (30.3068, 23.1952) centre (30.1946, 23.3075) ccw
  arc A4888 (33.1323, 23.3459) -> (32.9077, 23.1214) centre (33.02, 23.2336) ccw
  line L1777 (29.7901, 23.0596) -> (30.0021, 23.1676)
  arc A4889 (37.7177, 23.0759) -> (37.9422, 22.8514) centre (37.83, 22.9637) ccw
  arc A4890 (29.5148, 23.1371) -> (29.613, 22.8351) centre (29.5639, 22.9861) ccw
  arc A4891 (35.7178, 22.8514) -> (35.9423, 23.0759) centre (35.83, 22.9637) ccw
  line L1778 (29.7901, 27.7404) -> (29.5639, 27.8139)
  arc A4892 (30.8108, 23.1103) -> (30.6893, 22.817) centre (30.7501, 22.9637) ccw
  line L1779 (29.21, 22.9489) -> (29.3289, 22.9489)
  line L1780 (37.83, 22.9637) -> (38.3265, 23.4602)
  arc A4893 (36.4789, 22.8537) -> (36.4789, 22.5361) centre (36.4789, 22.6949) ccw
  arc A4894 (35.6723, 23.3459) -> (35.4477, 23.1214) centre (35.56, 23.2336) ccw
  arc A4895 (29.21, 23.1077) -> (29.21, 22.7902) centre (29.21, 22.9489) ccw
  arc A4896 (32.1011, 22.5361) -> (32.1011, 22.8537) centre (32.1011, 22.6949) ccw
  arc A4897 (33.8781, 22.5482) -> (33.9996, 22.8416) centre (33.9389, 22.6949) ccw
  line L1781 (35.83, 22.9637) -> (36.4789, 22.6949)
  arc A4898 (29.3688, 25.4) -> (29.0513, 25.4) centre (29.2101, 25.4) ccw
  line L1782 (29.3289, 22.9489) -> (29.5639, 22.9861)
  line L1783 (36.4789, 22.6949) -> (37.1811, 22.6949)
  arc A4899 (37.9422, 27.9486) -> (37.7177, 27.7241) centre (37.83, 27.8363) ccw
  arc A4900 (29.8392, 22.9086) -> (29.7411, 23.2106) centre (29.7902, 23.0596) ccw
  arc A4901 (38.1799, 23.521) -> (38.4732, 23.3995) centre (38.3266, 23.4603) ccw
  line L1784 (32.1011, 22.6949) -> (32.75, 22.9637)
  arc A4902 (33.1778, 22.8514) -> (33.4023, 23.0759) centre (33.2901, 22.9637) ccw
  line L1785 (35.56, 27.5663) -> (35.29, 27.8363)
  arc A4903 (29.8622, 27.8818) -> (29.7181, 27.5989) centre (29.7902, 27.7403) ccw
  line L1786 (28.4134, 29.337) -> (38.3274, 29.337)
  line L1787 (29.21, 25.4) -> (29.21, 27.8511)
  line L1788 (29.21, 27.8511) -> (29.0911, 27.8511)
  arc A4904 (28.3458, 27.7738) -> (28.49, 27.4909) centre (28.4179, 27.6324) ccw
  arc A4905 (30.3068, 27.6048) -> (30.0823, 27.3803) centre (30.1946, 27.4926) ccw
  arc A4906 (29.21, 28.0098) -> (29.21, 27.6923) centre (29.21, 27.8511) ccw
  line L1789 (32.75, 27.8363) -> (32.1011, 28.1051)
  arc A4907 (31.3989, 28.2638) -> (31.3989, 27.9463) centre (31.3989, 28.1051) ccw
  arc A4908 (28.1321, 27.621) -> (28.3188, 27.3641) centre (28.2254, 27.4926) ccw
  arc A4909 (33.9996, 27.9584) -> (33.8781, 28.2518) centre (33.9388, 28.1051) ccw
  arc A4910 (27.9253, 27.8056) -> (27.7007, 27.5811) centre (27.813, 27.6933) ccw
  arc A4911 (38.6352, 29.6233) -> (38.8597, 29.3988) centre (38.7475, 29.5111) ccw
  arc A4912 (29.0512, 25.4) -> (29.3687, 25.4) centre (29.2099, 25.4) ccw
  line L1790 (29.0911, 27.8511) -> (28.8561, 27.8139)
  arc A4913 (32.9077, 27.6786) -> (33.1323, 27.4541) centre (33.02, 27.5663) ccw
  arc A4914 (35.4022, 27.9486) -> (35.1777, 27.7241) centre (35.29, 27.8364) ccw
  line L1791 (35.29, 27.8363) -> (34.6411, 28.1051)
  arc A4915 (38.742, 24.0483) -> (38.4486, 24.1698) centre (38.5953, 24.109) ccw
  line L1792 (30.75, 27.8363) -> (30.3004, 27.3867)
  line L1793 (28.4179, 27.6324) -> (28.2255, 27.4926)
  arc A4916 (39.9906, 29.5638) -> (39.8691, 29.2705) centre (39.9299, 29.4172) ccw
  arc A4917 (40.3299, 29.0796) -> (40.4514, 29.373) centre (40.3907, 29.2263) ccw
  line L1794 (29.5639, 27.8139) -> (29.3289, 27.8511)
  arc A4918 (29.21, 25.2413) -> (29.21, 25.5588) centre (29.21, 25.4001) ccw
  arc A4919 (28.5808, 27.8914) -> (28.6789, 27.5894) centre (28.6299, 27.7404) ccw
  arc A4920 (29.7411, 27.5894) -> (29.8392, 27.8914) centre (29.7902, 27.7404) ccw
  line L1795 (27.813, 28.7366) -> (28.4134, 29.337)
  arc A4921 (33.2293, 27.983) -> (33.3508, 27.6897) centre (33.2901, 27.8363) ccw
  arc A4922 (30.1012, 27.3641) -> (30.2879, 27.621) centre (30.1946, 27.4926) ccw
  line L1796 (31.3989, 28.1051) -> (30.75, 27.8363)
  arc A4923 (38.2143, 27.2275) -> (38.4388, 27.452) centre (38.3266, 27.3398) ccw
  arc A4924 (34.6411, 27.9463) -> (34.6411, 28.2638) centre (34.6411, 28.1051) ccw
  arc A4925 (28.7019, 27.5989) -> (28.5578, 27.8818) centre (28.6299, 27.7404) ccw
  line L1797 (35.83, 27.8363) -> (35.56, 27.5663)
  arc A4926 (32.1619, 28.2518) -> (32.0404, 27.9584) centre (32.1012, 28.1051) ccw
  line L1798 (34.6411, 28.1051) -> (33.9389, 28.1051)
  arc A4927 (35.4477, 27.6786) -> (35.6723, 27.4541) centre (35.56, 27.5663) ccw
  arc A4928 (31.4596, 27.9584) -> (31.3381, 28.2518) centre (31.3988, 28.1051) ccw
  line L1799 (30.1945, 27.4926) -> (30.0021, 27.6324)
  arc A4929 (35.9423, 27.7241) -> (35.7178, 27.9486) centre (35.8301, 27.8364) ccw
  arc A4930 (38.754, 26.6909) -> (38.4365, 26.6909) centre (38.5953, 26.6909) ccw
  arc A4931 (38.4486, 26.6302) -> (38.742, 26.7517) centre (38.5953, 26.6909) ccw
  line L1800 (33.02, 27.5663) -> (32.75, 27.8363)
  arc A4932 (38.4365, 24.1091) -> (38.754, 24.1091) centre (38.5953, 24.1091) ccw
  arc A4933 (34.7019, 28.2518) -> (34.5804, 27.9584) centre (34.6412, 28.1051) ccw
  arc A4934 (35.7693, 27.983) -> (35.8908, 27.6897) centre (35.8301, 27.8363) ccw
  arc A4935 (30.6893, 27.983) -> (30.8108, 27.6897) centre (30.7501, 27.8364) ccw
  arc A4936 (30.1881, 27.499) -> (30.4126, 27.2744) centre (30.3003, 27.3867) ccw
  arc A4937 (32.1011, 27.9463) -> (32.1011, 28.2638) centre (32.1011, 28.1051) ccw
  arc A4938 (36.4789, 28.2638) -> (36.4789, 27.9463) centre (36.4789, 28.1051) ccw
  line L1801 (38.3265, 23.4602) -> (38.5953, 24.1091)
  line L1802 (30.3004, 27.3867) -> (30.1945, 27.4926)
  arc A4939 (32.6892, 27.6897) -> (32.8107, 27.983) centre (32.7499, 27.8364) ccw
  arc A4940 (30.1881, 27.2744) -> (30.4126, 27.499) centre (30.3004, 27.3867) ccw
  line L1803 (37.83, 27.8363) -> (37.1811, 28.1051)
  line L1804 (37.1811, 28.1051) -> (36.4789, 28.1051)
  line L1805 (38.5953, 26.6909) -> (38.3265, 27.3398)
  arc A4941 (30.8623, 27.7241) -> (30.6378, 27.9486) centre (30.7501, 27.8364) ccw
  arc A4942 (37.7692, 27.6897) -> (37.8907, 27.983) centre (37.83, 27.8364) ccw
  arc A4943 (38.4732, 27.4005) -> (38.1799, 27.279) centre (38.3265, 27.3398) ccw
  line L1806 (32.1011, 28.1051) -> (31.3989, 28.1051)
  arc A4944 (37.2419, 28.2518) -> (37.1204, 27.9584) centre (37.1812, 28.1051) ccw
  line L1807 (39.41, 30.1735) -> (39.5772, 29.7698)
  arc A4945 (29.3688, 27.8511) -> (29.0513, 27.8511) centre (29.2101, 27.8511) ccw
  arc A4946 (39.8176, 29.3049) -> (40.0421, 29.5294) centre (39.9299, 29.4172) ccw
  arc A4947 (29.5391, 27.6571) -> (29.5887, 27.9707) centre (29.5639, 27.8139) ccw
  line L1808 (27.813, 27.6933) -> (27.813, 28.7366)
  line L1809 (28.8561, 27.8139) -> (28.6299, 27.7404)
  arc A4948 (28.0073, 27.499) -> (28.2319, 27.2744) centre (28.1196, 27.3867) ccw
  arc A4949 (28.5257, 29.2247) -> (28.3012, 29.4493) centre (28.4135, 29.337) ccw
  line L1810 (39.5772, 29.7698) -> (39.9298, 29.4172)
  arc A4950 (29.3687, 27.8511) -> (29.0512, 27.8511) centre (29.2099, 27.8511) ccw
  arc A4951 (29.613, 27.9649) -> (29.5148, 27.6629) centre (29.5639, 27.8139) ccw
  arc A4952 (38.8082, 29.3643) -> (38.6867, 29.6577) centre (38.7475, 29.511) ccw
  arc A4953 (28.0073, 27.2744) -> (28.2319, 27.499) centre (28.1196, 27.3867) ccw
  arc A4954 (27.7007, 28.8488) -> (27.9253, 28.6243) centre (27.813, 28.7366) ccw
  arc A4955 (28.8313, 27.9707) -> (28.8809, 27.6571) centre (28.8561, 27.8139) ccw
  arc A4956 (29.1159, 27.6943) -> (29.0662, 28.0079) centre (29.091, 27.8511) ccw
  arc A4957 (29.21, 25.5588) -> (29.21, 25.2413) centre (29.21, 25.4001) ccw
  line L1811 (28.2255, 27.4926) -> (28.1196, 27.3867)
  arc A4958 (29.21, 27.6923) -> (29.21, 28.0098) centre (29.21, 27.8511) ccw
  line L1812 (28.6299, 27.7404) -> (28.4179, 27.6324)
  line L1813 (38.3274, 29.337) -> (38.7475, 29.511)
  arc A4959 (38.3274, 29.1782) -> (38.3274, 29.4958) centre (38.3274, 29.337) ccw
  arc A4960 (28.3377, 27.3803) -> (28.1132, 27.6048) centre (28.2255, 27.4926) ccw
  arc A4961 (28.5112, 27.5039) -> (28.3246, 27.7608) centre (28.4179, 27.6324) ccw
  arc A4962 (27.6542, 27.6933) -> (27.9717, 27.6933) centre (27.813, 27.6933) ccw
  arc A4963 (29.0513, 25.4) -> (29.3688, 25.4) centre (29.2101, 25.4) ccw
  line L1814 (29.21, 27.8511) -> (29.21, 25.4)
  arc A4964 (28.9052, 27.6629) -> (28.807, 27.9649) centre (28.8561, 27.8139) ccw
  arc A4965 (39.5222, 30.0613) -> (39.2977, 30.2858) centre (39.41, 30.1736) ccw
  arc A4966 (28.4134, 29.4958) -> (28.4134, 29.1782) centre (28.4134, 29.337) ccw
  arc A4967 (51.943, 28.7338) -> (51.943, 28.4163) centre (51.943, 28.5751) ccw
  arc A4968 (5.5245, 29.0512) -> (5.5245, 29.3688) centre (5.5245, 29.21) ccw
  arc A4969 (32.4997, 28.0988) -> (32.4997, 27.7813) centre (32.4997, 27.9401) ccw
  arc A4970 (35.0397, 28.0988) -> (35.0397, 27.7813) centre (35.0397, 27.9401) ccw
  arc A4971 (56.8579, 27.4638) -> (56.8579, 27.1462) centre (56.8579, 27.305) ccw
  arc A4972 (9.7155, 30.0038) -> (9.7155, 29.6863) centre (9.7155, 29.8451) ccw
  arc A4973 (71.628, 26.8288) -> (71.628, 26.5113) centre (71.628, 26.67) ccw
  arc A4974 (74.803, 29.3688) -> (74.803, 29.0512) centre (74.803, 29.21) ccw
  arc A4975 (0.7747, 27.4638) -> (0.7747, 27.1462) centre (0.7747, 27.305) ccw
  arc A4976 (63.7886, 27.1462) -> (63.7886, 27.4638) centre (63.7886, 27.305) ccw
  arc A4977 (38.3409, 27.4638) -> (38.3409, 27.1462) centre (38.3409, 27.305) ccw
  arc A4978 (59.449, 29.6863) -> (59.449, 30.0038) centre (59.449, 29.8451) ccw
  arc A4979 (54.9021, 29.0512) -> (54.9021, 29.3688) centre (54.9021, 29.21) ccw
  arc A4980 (56.8579, 26.8288) -> (56.8579, 26.5113) centre (56.8579, 26.67) ccw
  arc A4981 (0.7747, 28.0988) -> (0.7747, 27.7813) centre (0.7747, 27.9401) ccw
  arc A4982 (59.2514, 26.8288) -> (59.2514, 26.5113) centre (59.2514, 26.67) ccw
  arc A4983 (62.357, 29.0512) -> (62.357, 29.3688) centre (62.357, 29.21) ccw
  arc A4984 (76.9497, 29.3688) -> (76.9497, 29.0512) centre (76.9497, 29.21) ccw
  arc A4985 (72.0436, 29.0512) -> (72.0436, 29.3688) centre (72.0436, 29.21) ccw
  arc A4986 (74.0064, 28.0988) -> (74.0064, 27.7813) centre (74.0064, 27.9401) ccw
  arc A4987 (62.5258, 28.4163) -> (62.5258, 28.7338) centre (62.5258, 28.5751) ccw
  arc A4988 (6.5615, 27.1462) -> (6.5615, 27.4638) centre (6.5615, 27.305) ccw
  arc A4989 (53.34, 26.8288) -> (53.34, 26.5113) centre (53.34, 26.67) ccw
  arc A4990 (53.34, 27.1462) -> (53.34, 27.4638) centre (53.34, 27.305) ccw
  arc A4991 (84.2253, 29.0512) -> (84.2253, 29.3688) centre (84.2253, 29.21) ccw
  arc A4992 (9.7155, 29.3688) -> (9.7155, 29.0512) centre (9.7155, 29.21) ccw
  arc A4993 (84.2253, 28.4163) -> (84.2253, 28.7338) centre (84.2253, 28.5751) ccw
  arc A4994 (54.5068, 27.4638) -> (54.5068, 27.1462) centre (54.5068, 27.305) ccw
  arc A4995 (5.5245, 28.4163) -> (5.5245, 28.7338) centre (5.5245, 28.5751) ccw
  arc A4996 (56.8579, 30.0038) -> (56.8579, 29.6863) centre (56.8579, 29.8451) ccw
  arc A4997 (31.0003, 27.7813) -> (31.0003, 28.0988) centre (31.0003, 27.9401) ccw
  arc A4998 (54.9021, 27.1462) -> (54.9021, 27.4638) centre (54.9021, 27.305) ccw
  arc A4999 (54.8178, 26.8288) -> (54.8178, 26.5113) centre (54.8178, 26.67) ccw
  arc A5000 (29.21, 27.4638) -> (29.21, 27.1462) centre (29.21, 27.305) ccw
  arc A5001 (74.6341, 28.7338) -> (74.6341, 28.4163) centre (74.6341, 28.5751) ccw
  arc A5002 (56.8579, 29.3688) -> (56.8579, 29.0512) centre (56.8579, 29.21) ccw
  arc A5003 (39.546, 29.6863) -> (39.546, 30.0038) centre (39.546, 29.8451) ccw
  arc A5004 (23.671, 29.6863) -> (23.671, 30.0038) centre (23.671, 29.8451) ccw
  arc A5005 (60.2103, 29.0512) -> (60.2103, 29.3688) centre (60.2103, 29.21) ccw
  arc A5006 (51.943, 29.3688) -> (51.943, 29.0512) centre (51.943, 29.21) ccw
  arc A5007 (72.1491, 29.6863) -> (72.1491, 30.0038) centre (72.1491, 29.8451) ccw
  arc A5008 (67.2068, 30.0038) -> (67.2068, 29.6863) centre (67.2068, 29.8451) ccw
  arc A5009 (0.7747, 28.7338) -> (0.7747, 28.4163) centre (0.7747, 28.5751) ccw
  arc A5010 (75.4503, 29.0512) -> (75.4503, 29.3688) centre (75.4503, 29.21) ccw
  arc A5011 (61.7097, 29.3688) -> (61.7097, 29.0512) centre (61.7097, 29.21) ccw
  arc A5012 (66.04, 30.9563) -> (66.04, 31.2738) centre (66.04, 31.1151) ccw
  arc A5013 (81.28, 30.6388) -> (81.28, 30.3212) centre (81.28, 30.48) ccw
  arc A5014 (71.8947, 30.3212) -> (71.8947, 30.6388) centre (71.8947, 30.48) ccw
  arc A5015 (65.1164, 29.3688) -> (65.1164, 29.0512) centre (65.1164, 29.21) ccw
  arc A5016 (12.333, 29.6863) -> (12.333, 30.0038) centre (12.333, 29.8451) ccw
  arc A5017 (77.9903, 29.0512) -> (77.9903, 29.3688) centre (77.9903, 29.21) ccw
  arc A5018 (56.8579, 28.7338) -> (56.8579, 28.4163) centre (56.8579, 28.5751) ccw
  arc A5019 (23.382, 29.0512) -> (23.382, 29.3688) centre (23.382, 29.21) ccw
  arc A5020 (54.9021, 29.6863) -> (54.9021, 30.0038) centre (54.9021, 29.8451) ccw
  arc A5021 (16.623, 30.6388) -> (16.623, 30.3212) centre (16.623, 30.48) ccw
  arc A5022 (67.5513, 31.2738) -> (67.5513, 30.9563) centre (67.5513, 31.1151) ccw
  arc A5023 (81.28, 30.3212) -> (81.28, 30.6388) centre (81.28, 30.48) ccw
  arc A5024 (51.1464, 30.6388) -> (51.1464, 30.3212) centre (51.1464, 30.48) ccw
  arc A5025 (11.698, 30.3212) -> (11.698, 30.6388) centre (11.698, 30.48) ccw
  arc A5026 (79.4897, 29.3688) -> (79.4897, 29.0512) centre (79.4897, 29.21) ccw
  arc A5027 (15.988, 30.0038) -> (15.988, 29.6863) centre (15.988, 29.8451) ccw
  arc A5028 (54.9021, 28.4163) -> (54.9021, 28.7338) centre (54.9021, 28.5751) ccw
  arc A5029 (81.28, 30.9563) -> (81.28, 31.2738) centre (81.28, 31.1151) ccw
  arc A5030 (51.7742, 30.0038) -> (51.7742, 29.6863) centre (51.7742, 29.8451) ccw
  arc A5031 (82.4468, 30.0038) -> (82.4468, 29.6863) centre (82.4468, 29.8451) ccw
  arc A5032 (27.813, 28.7338) -> (27.813, 28.4163) centre (27.813, 28.5751) ccw
  arc A5033 (41.162, 28.4163) -> (41.162, 28.7338) centre (41.162, 28.5751) ccw
  arc A5034 (0.7747, 29.3688) -> (0.7747, 29.0512) centre (0.7747, 29.21) ccw
  arc A5035 (26.3236, 30.3212) -> (26.3236, 30.6388) centre (26.3236, 30.48) ccw
  arc A5036 (81.28, 30.0038) -> (81.28, 29.6863) centre (81.28, 29.8451) ccw
  arc A5037 (56.8579, 30.6388) -> (56.8579, 30.3212) centre (56.8579, 30.48) ccw
  arc A5038 (0.7747, 30.0038) -> (0.7747, 29.6863) centre (0.7747, 29.8451) ccw
  arc A5039 (28.2864, 29.3688) -> (28.2864, 29.0512) centre (28.2864, 29.21) ccw
  arc A5040 (39.0814, 30.0038) -> (39.0814, 29.6863) centre (39.0814, 29.8451) ccw
  arc A5041 (40.527, 29.0512) -> (40.527, 29.3688) centre (40.527, 29.21) ccw
  arc A5042 (5.5245, 29.6863) -> (5.5245, 30.0038) centre (5.5245, 29.8451) ccw
  arc A5043 (84.2253, 30.9563) -> (84.2253, 31.2738) centre (84.2253, 31.1151) ccw
  arc A5044 (5.9265, 30.3212) -> (5.9265, 30.6388) centre (5.9265, 30.48) ccw
  arc A5045 (15.4025, 33.1788) -> (15.4025, 32.8613) centre (15.4025, 33.0201) ccw
  arc A5046 (6.5615, 30.9563) -> (6.5615, 31.2738) centre (6.5615, 31.1151) ccw
  arc A5047 (54.9021, 30.3212) -> (54.9021, 30.6388) centre (54.9021, 30.48) ccw
  arc A5048 (0.7747, 30.6388) -> (0.7747, 30.3212) centre (0.7747, 30.48) ccw
  arc A5049 (8.6785, 31.2738) -> (8.6785, 30.9563) centre (8.6785, 31.1151) ccw
  arc A5050 (81.28, 29.6863) -> (81.28, 30.0038) centre (81.28, 29.8451) ccw
  arc A5051 (54.9021, 30.9563) -> (54.9021, 31.2738) centre (54.9021, 31.1151) ccw
  arc A5052 (66.04, 30.3212) -> (66.04, 30.6388) centre (66.04, 30.48) ccw
  arc A5053 (82.7578, 30.6388) -> (82.7578, 30.3212) centre (82.7578, 30.48) ccw
  arc A5054 (11.063, 30.9563) -> (11.063, 31.2738) centre (11.063, 31.1151) ccw
  arc A5055 (81.28, 31.9088) -> (81.28, 31.5912) centre (81.28, 31.75) ccw
  arc A5056 (51.6314, 31.9088) -> (51.6314, 31.5912) centre (51.6314, 31.75) ccw
  arc A5057 (66.04, 29.6863) -> (66.04, 30.0038) centre (66.04, 29.8451) ccw
  arc A5058 (59.1947, 30.3212) -> (59.1947, 30.6388) centre (59.1947, 30.48) ccw
  arc A5059 (59.1947, 30.9563) -> (59.1947, 31.2738) centre (59.1947, 31.1151) ccw
  arc A5060 (11.924, 33.1788) -> (11.924, 32.8613) centre (11.924, 33.0201) ccw
  arc A5061 (0.7747, 32.5437) -> (0.7747, 32.2263) centre (0.7747, 32.385) ccw
  arc A5062 (15.7861, 32.8613) -> (15.7861, 33.1788) centre (15.7861, 33.0201) ccw
  arc A5063 (56.8579, 31.2738) -> (56.8579, 30.9563) centre (56.8579, 31.1151) ccw
  arc A5064 (82.7913, 31.2738) -> (82.7913, 30.9563) centre (82.7913, 31.1151) ccw
  arc A5065 (17.258, 31.2738) -> (17.258, 30.9563) centre (17.258, 31.1151) ccw
  arc A5066 (14.6382, 32.5437) -> (14.6382, 32.2263) centre (14.6382, 32.385) ccw
  arc A5067 (13.3018, 32.2263) -> (13.3018, 32.5437) centre (13.3018, 32.385) ccw
  arc A5068 (66.04, 31.2738) -> (66.04, 30.9563) centre (66.04, 31.1151) ccw
  arc A5069 (54.9021, 31.5912) -> (54.9021, 31.9088) centre (54.9021, 31.75) ccw
  arc A5070 (82.7913, 32.5437) -> (82.7913, 32.2263) centre (82.7913, 32.385) ccw